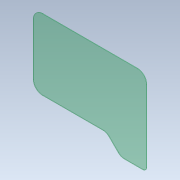
# Autodesk Inventor part: Стекло
Saved by Autodesk Inventor 2021.2 (Build 252289000, 289)
## iProperties
Created: 2022-11-29
Part Number: Стекло
Material: Типовые
Document SubType Name: ЛистМат
Designer: Voodoo
Density: 1 g/cm^3
Sheet Metal Rule: По умолчанию_мм
Appearance: Прозрачный — зеленый 1
Mass: 71.0705 g
Surface Area: 761.316 cm^2
Volume: 71.0705 cm^3
Flat Pattern Width: 29.8 cm
Flat Pattern Length: 39.7 cm
Flat Pattern Area: 1183.06 cm^2
Sheet Metal Width: 298,000 мм
Sheet Metal Length: 397,000 мм
Sheet Metal Area: 118306,000 мм^2
Author: Voodoo
Autodesk Inventor part; units mm, degrees
ref_plane "YZ Plane" through (0, 0, 0) normal (1, 0, 0) x (0, 1, 0)
ref_plane "XZ Plane" through (0, 0, 0) normal (0, 1, 0) x (-1, 0, 0)
ref_plane "XY Plane" through (0, 0, 0) normal (0, 0, 1) x (1, 0, 0)
sketch "Эскиз1" plane through (0, 0, 0) normal (0, 0, 1) x (1, 0, 0)
  line L0 (-166.5, -124) -> (46.0736, -124)
  line L1 (198.5, -124) -> (198.5, 92)
  line L2 (166.5, 124) -> (-166.5, 124)
  line L3 (-198.5, 92) -> (-198.5, -92)
  line L4 (-198.5, -124) -> (198.5, 124) construction
  line L5 (198.5, -124) -> (-198.5, 124) construction
  arc A0 (-166.5, 124) -> (-198.5, 92) centre (-166.5, 92) ccw
  arc A1 (198.5, 92) -> (166.5, 124) centre (166.5, 92) ccw
  arc A2 (-198.5, -92) -> (-166.5, -124) centre (-166.5, -92) ccw
  line L6 (198.5, -124) -> (198.5, -162)
  line L7 (186.5, -174) -> (120.9264, -174)
  line L8 (99.7132, -165.2132) -> (67.2868, -132.7868)
  arc A3 (186.5, -174) -> (198.5, -162) centre (186.5, -162) ccw
  arc A4 (99.7132, -165.2132) -> (120.9264, -174) centre (120.9264, -144) ccw
  arc A5 (67.2868, -132.7868) -> (46.0736, -124) centre (46.0736, -154) ccw
  point P0 (0, 0)
  point P1 (198.5, -174)
  point P2 (108.5, -174)
  dimension "d2" = 397
  dimension "d3" = 248
  dimension "d4" = 32
  dimension "d5" = 298
  dimension "d6" = 12
  dimension "d7" = 50
  dimension "d8" = 90
  dimension "d9" = 135
  dimension "d10" = 30
  measures "d2" distance of L5.end L4.end
  measures "d3" distance of L4.end L1.start
  measures "d4" radius of A0
  measures "d5" distance between parallel lines of L7 L2
  measures "d6" radius of A3
  measures "d7" distance between parallel lines of L0 L7
  measures "d8" distance from line of L6 point (108.5, -174)
  measures "d9" angle of L0 L8
  measures "d10" radius of A4
extrude "Пластина1" add sketch "Эскиз1" along normal blind 2
sketch "Эскиз5" plane through (0, 0, 2) normal (0, 0, 1) x (1, 0, 0)
  line L0 (198.5, 92) -> (198.5, -162) projected
  arc A0 (198.5, 92) -> (166.5, 124) centre (166.5, 92) ccw projected
  line L1 (-166.5, 124) -> (166.5, 124) projected
  arc A1 (-166.5, 124) -> (-198.5, 92) centre (-166.5, 92) ccw projected
  line L2 (-198.5, -92) -> (-198.5, 92) projected
  arc A2 (-198.5, -92) -> (-166.5, -124) centre (-166.5, -92) ccw projected
  line L3 (46.0736, -124) -> (-166.5, -124) projected
  arc A3 (67.2868, -132.7868) -> (46.0736, -124) centre (46.0736, -154) ccw projected
  line L4 (99.7132, -165.2132) -> (67.2868, -132.7868) projected
  arc A4 (99.7132, -165.2132) -> (120.9264, -174) centre (120.9264, -144) ccw projected
  line L5 (186.5, -174) -> (120.9264, -174) projected
  arc A5 (186.5, -174) -> (198.5, -162) centre (186.5, -162) ccw projected
  circle A6 centre (154.5, -142) radius 25
  line L6 (-172, 97.5) -> (172, 97.5)
  line L7 (172, 97.5) -> (172, -94.5)
  line L8 (172, -94.5) -> (-172, -94.5)
  line L9 (-172, -94.5) -> (-172, 97.5)
  point P0 (0, 0)
  dimension "d57" = 50
  dimension "d58" = 26.5
  dimension "d59" = 26.5
  dimension "d60" = 26.5
  dimension "d61" = 29.5
  dimension "d62" = 44
  dimension "d63" = 32
  constraints: 8 end point, 2 parallel, 1 centre point, 1 horizontal, 1 perpendicular
  measures "d57" diameter of A6
  measures "d58" distance between parallel lines of L1 L6
  measures "d59" distance between parallel lines of L2 L9
  measures "d60" distance between parallel lines of L0 L7
  measures "d61" distance between parallel lines of L3 L8
  measures "d62" distance from line of L0 A6.centre
  measures "d63" distance from line of A6.centre L5
extrude "Вырез4" cut sketch "Эскиз5" against normal blind 2 contours A6 | L6 L7 L8 L9
fillet "УглСкругление1" radius 6 4 edges at (-172, 97.5, 1) (172, 97.5, 1) (172, -94.5, 1) (-172, -94.5, 1)
equation "\"d59\" = d60"
equation "\"d64\" = Толщина"
equation "\"d12\" = Толщина"
equation "\"Радиус_гибки\" = Толщина"
equation "\"Ширина_просечки\" = Толщина"
equation "\"Глубина_просечки\" = 0.5 * Толщина"
equation "\"Размер_просечки\" = 4 * Толщина"
equation "\"Мин_остаток\" = 2 * Толщина"
equation "\"Радиус_перехода\" = Радиус_гибки"
equation "\"Радиус_Якоби\" = Радиус_гибки"
equation "\"Размер_зазора\" = Толщина"
equation "\"Толщина\" = 2"
